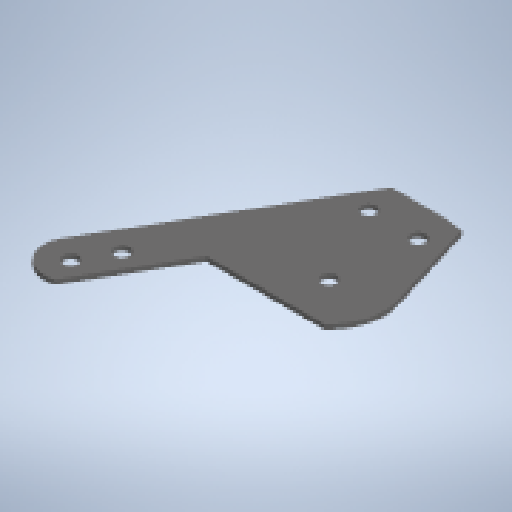
# Autodesk Inventor part: screw_cover_upper
Saved by Autodesk Inventor 2024.1 (Build 281209000, 209)
## iProperties
Created: 2025-01-18
Part Number: screw_cover_upper
Material: 一般
Document SubType Name: Modeling
Designer: hibik
Density: 1 g/cm^3
Appearance: 既定
Author: hibik
Autodesk Inventor part; units mm, degrees
ref_plane "YZ Plane" through (0, 0, 0) normal (1, 0, 0) x (0, 1, 0)
ref_plane "XZ Plane" through (0, 0, 0) normal (0, 1, 0) x (-1, 0, 0)
sketch "スケッチ1" plane through (0, 0, 0) normal (0, 1, 0) x (-1, 0, 0)
  circle A0 centre (0, 0) radius 8.9
  line L0 (0, -8.9) -> (63.2748, -8.9)
  line L1 (63.2748, -8.9) -> (63.2748, 8.9)
  line L2 (63.2748, 8.9) -> (0, 8.9)
  line L3 (0, 8.9) -> (0, -8.9)
  circle A1 centre (0, 0) radius 8.4
  line L4 (0, -8.4) -> (63.2748, -8.4)
  line L5 (63.2748, -8.4) -> (63.2748, 8.4)
  line L6 (63.2748, 8.4) -> (0, 8.4)
  line L7 (0, 8.4) -> (0, -8.4)
  point P0 (0, 8.4)
  point P1 (0, 8.9)
  dimension "d0" = 17.8
  dimension "d1" = 16.8
  constraints: 16 end point, 6 horizontal, 4 parallel, 3 coincident, 2 perpendicular, 1 collinear, 6 other
extrude "押し出し1" add sketch "スケッチ1" along normal blind 0.85 contours L3 A1 A0 | L2 L1 L6 A0 | A0 L6 L3 | L3 L4 A0 | A0 L4 L1 L0
sketch "スケッチ2" plane through (0, 0.85, 0) normal (0, 1, 0) x (1, 0, 0)
  circle A0 centre (0, 0) radius 12
  line L0 (0, 12) -> (-63.2748, 12)
  line L1 (-63.2748, 12) -> (-63.2748, -12)
  line L2 (-63.2748, -12) -> (0, -12)
  line L3 (0, -12) -> (0, 12)
  line L4 (-63.2748, 8.9) -> (-63.2748, 8.4) projected
  line L5 (-63.2748, 8.4) -> (0, 8.4) projected
  line L6 (0, -8.4) -> (-63.2748, -8.4) projected
  arc A1 (0, -8.4) -> (0, 8.4) centre (0, 0) ccw projected
  point P0 (0, -12)
  dimension "d4" = 24
  constraints: 8 end point, 3 horizontal, 2 parallel, 1 coincident, 1 collinear, 1 perpendicular, 3 other
extrude "押し出し2" add sketch "スケッチ2" along normal blind 1 contours A0 L3 A1 | L3 L5 A0 | A0 L5 L1 L0 | L2 L1 L6 A0 | A0 L6 L3
mirror "ミラー1" about plane through (-27.1874, 0, 0) normal (0, -1, 0)
sketch "スケッチ3" plane through (0, 1.85, 0) normal (0, 1, 0) x (1, 0, 0)
  line L0 (-14.7409, 17.0236) -> (-35.8476, -19.5343) projected
  line L1 (0, -8.4) -> (-63.2748, -8.4) projected
  line L2 (-63.2748, -8.4) -> (-63.2748, -12) projected
  line L3 (-63.2748, -12) -> (0, -12) projected
  arc A0 (0, -12) -> (0, 12) centre (0, 0) ccw projected
  line L4 (0, 12) -> (-63.2748, 12) projected
  line L5 (-63.2748, 12) -> (-63.2748, 8.4) projected
  line L6 (-63.2748, 8.4) -> (0, 8.4) projected
  arc A1 (0, -8.4) -> (0, 8.4) centre (0, 0) ccw projected
  point P0 (-31.4977, -12)
  point P1 (-29.4192, -8.4)
  point P2 (-19.7197, 8.4)
  point P3 (-17.6412, 12)
extrude "押し出し3" cut sketch "スケッチ3" against normal through all contours L0 L6 L5 L4 | L0 L3 L2 L1
ref_plane "作業平面1" through (0, -0.65, 0) normal (0, 1, 0) x (1, 0, 0)
sketch "スケッチ4" plane through (0, -0.65, 0) normal (0, 1, 0) x (1, 0, 0)
  line L0 (-19.7197, 8.4) -> (0, 8.4) projected
  arc A0 (0, -8.4) -> (0, 8.4) centre (0, 0) ccw projected
  line L1 (0, -8.4) -> (-29.4192, -8.4) projected
  line L2 (-19.7197, 8.4) -> (-29.4192, -8.4)
  circle A1 centre (0, 0) radius 1.6
  dimension "d10" = 3.2
  constraints: 2 coincident, 2 end point, 1 centre point
  measures "d10" diameter of A1
extrude "押し出し4" add sketch "スケッチ4" along normal up to surface (2.5 mm away)
fillet "フィレット1" radius 1 3 edges at (-9.8599, -0.65, -8.4) (8.4, -0.65, 0) (-14.7096, -0.65, 8.4)
sketch "スケッチ5" plane through (0, 1.85, 0) normal (0, 1, 0) x (1, 0, 0)
  circle A0 centre (-27.8315, -17.35) radius 1.6 projected
  circle A1 centre (-8.7282, 17.4379) radius 1.6 projected
  line L0 (0, 12) -> (-17.6412, 12) projected
  line L1 (-17.6412, 12) -> (-10.5885, 24.2158)
  line L2 (-10.5885, 24.2158) -> (0, 24.2158)
  line L3 (-39.933, -26.6105) -> (-10.6554, 24.0998) projected
  line L4 (0, 12) -> (-17.6412, 12) projected
  circle A2 centre (0, 0) radius 24.2158
  arc A3 (0, -12) -> (0, 12) centre (0, 0) ccw projected
  line L5 (11.4695, 3.5285) -> (5.2849, 23.6321)
  circle A4 centre (1.9592, 17.4379) radius 1.6
  line L6 (-39.933, -26.6105) -> (-10.6554, 24.0998) projected
  circle A5 centre (-31.9338, -24.4553) radius 1.6 projected
  circle A6 centre (-36, -34.6362) radius 1.6 projected
  circle A7 centre (-27.8315, -17.35) radius 1.6 projected
  line L7 (-39.933, -26.6105) -> (-10.6554, 24.0998) projected
  line L8 (-40, -50) -> (-40, -26.8605) projected
  line L9 (-38, -50.5) -> (-39.5, -50.5) projected
  line L10 (-31, -42) -> (-31, -32.0566) projected
  line L11 (-30.933, -31.8066) -> (-18.1986, -9.75) projected
  line L12 (-37.5, -50) -> (-37.5, -43) projected
  line L13 (-37, -42.5) -> (-31.5, -42.5) projected
  circle A8 centre (-31.9338, -24.4553) radius 5.85
  arc A9 (19.2639, -16.134) -> (19.9469, -15.951) centre (19.5139, -15.701) ccw projected
  line L14 (29.8557, 1.2115) -> (19.9469, -15.951) projected
  arc A10 (29.8557, 1.2115) -> (29.8557, 1.7115) centre (29.4226, 1.4615) ccw projected
  line L15 (10.25, 35.6695) -> (29.8557, 1.7115) projected
  arc A11 (10.25, 35.6695) -> (9.567, 35.8525) centre (9.817, 35.4195) ccw projected
  line L16 (-10.4724, 24.2828) -> (9.567, 35.8525) projected
  arc A12 (-10.4724, 24.2828) -> (-10.6554, 24.0998) centre (-10.2224, 23.8498) ccw projected
  arc A13 (-39.933, -26.6105) -> (-40, -26.8605) centre (-39.5, -26.8605) ccw projected
  arc A14 (-40, -50) -> (-39.5, -50.5) centre (-39.5, -50) ccw projected
  arc A15 (-38, -50.5) -> (-37.5, -50) centre (-38, -50) ccw projected
  arc A16 (-37, -42.5) -> (-37.5, -43) centre (-37, -43) ccw projected
  arc A17 (-31.5, -42.5) -> (-31, -42) centre (-31.5, -42) ccw projected
  arc A18 (-30.933, -31.8066) -> (-31, -32.0566) centre (-30.5, -32.0566) ccw projected
  arc A19 (-17.7656, -9.5) -> (-18.1986, -9.75) centre (-17.7656, -10) ccw projected
  line L17 (-17.7656, -9.5) -> (7.6395, -9.5) projected
  arc A20 (7.8895, -9.567) -> (7.6395, -9.5) centre (7.6395, -10) ccw projected
  line L18 (7.8895, -9.567) -> (19.2639, -16.134) projected
  circle A21 centre (1.9592, 17.4379) radius 1.6 projected
  circle A22 centre (24.5152, 1.2615) radius 1.6 projected
  circle A23 centre (5.1388, 27.5224) radius 1.6 projected
  circle A24 centre (13.1994, 17.561) radius 1.6 projected
  circle A25 centre (20.4199, -5.8317) radius 1.6 projected
  circle A26 centre (-8.7282, 17.4379) radius 1.6 projected
  circle A27 centre (0, 0) radius 1.5 projected
  point P0 (0, 24.2158)
  point P1 (-20.2427, -13.2905)
  point P2 (-12.6465, 20.6512)
  point P3 (-37, -21.5303)
  point P4 (-29.8432, -29.9191)
  point P5 (-26.1568, -23.5339)
  dimension "d14" = 15
  dimension "d15" = 3.2
  dimension "d16" = 5
  constraints: 4 end point, 3 centre point, 3 point on circle, 2 coincident, 2 tangent, 1 collinear, 1 horizontal, 1 horizontal alignment, 5 other
  measures "d14" distance from line of L1.end L5
  measures "d15" diameter of A4
  measures "d16" distance from line of L5 A4.centre
extrude "押し出し5" add sketch "スケッチ5" against normal blind 1 contours A1 | A3 L17 A19 L11 A2 L3 L0 | L0 L1 A2 L5 A3 | L5 A2 A22 L18 A20 L17 A3 | L1 A12 L2 A2 | A2 L11 A8 L3 | A2 L2 A12 L16 A11 L15 A10 L14 A9 L18 A22 | L1 L2 A12 | A8 L11 A18 L10 A17 L13 A16 L12 A15 L9 A14 L8 A13 L3 | A8 L11 | A22 A2 | A2 A22 | A8 L11 | A4 | A6 | A23 | A24 | A25 | A27
sketch "スケッチ6" plane through (0, 1.85, 0) normal (0, 1, 0) x (1, 0, 0)
  line L0 (-19.4977, -12) -> (0, -12) projected
  line L1 (-19.4977, -12) -> (-17.7656, -9)
  line L2 (-17.7656, -9) -> (7.9373, -9)
  arc A0 (0, -12) -> (0, 12) centre (0, 0) ccw projected
  line L3 (-29.8432, -29.9191) -> (-19.4977, -12) projected
  point P0 (-25.741, -22.8137)
  point P1 (-20.2427, -13.2905)
  point P2 (-31, -31.9226)
  dimension "d19" = 3
  constraints: 4 end point, 1 collinear, 1 parallel, 1 point on circle
  measures "d19" distance between parallel lines of L2 L0
extrude "押し出し6" cut sketch "スケッチ6" against normal through all
sketch "スケッチ7" plane through (0, -1.85, 0) normal (0, -1, 0) x (1, 0, 0)
  line L0 (-19.3733, -9) -> (0, -9) projected
  line L1 (-17.7656, 9) -> (-19.4977, 12) projected
  line L2 (-31.4977, 12) -> (-19.4977, 12) projected
  line L3 (-31.4977, 12) -> (-29.4192, 8.4) projected
  line L4 (0, 8.4) -> (-29.4192, 8.4) projected
  arc A0 (0, -8.4) -> (0, 8.4) centre (0, 0) ccw projected
  line L5 (-19.7197, -8.4) -> (0, -8.4) projected
  line L6 (-19.7197, -8.4) -> (-17.6412, -12) projected
  line L7 (0, -12) -> (-17.6412, -12) projected
  arc A1 (0, -12) -> (7.9373, 9) centre (0, 0) ccw projected
  line L8 (7.9373, 9) -> (-17.7656, 9) projected
  circle A2 centre (0, 0) radius 1.6 projected
  line L9 (0, -7.4) -> (-20.2971, -7.4) projected
  arc A3 (0, -7.4) -> (0, 7.4) centre (0, 0) ccw projected
  line L10 (-28.8418, 7.4) -> (0, 7.4) projected
  line L11 (-20.2971, -7.4) -> (-28.8418, 7.4) projected
  circle A4 centre (0, 0) radius 9 projected
  line L12 (-17.7656, 9) -> (7.9373, 9) projected
  line L13 (-10.5631, -24.2158) -> (-10.5885, -24.2158) projected
  arc A5 (-26.1568, 23.5339) -> (-29.8432, 29.9191) centre (-31.9338, 24.4553) ccw projected
  line L14 (-26.1568, 23.5339) -> (-17.7656, 9) projected
  circle A6 centre (-27.8315, 17.35) radius 1.6 projected
  circle A7 centre (-31.9338, 24.4553) radius 1.6 projected
  arc A8 (7.9373, 9) -> (7.3314, 9.5) centre (0, 0) ccw projected
  line L15 (7.3314, 9.5) -> (7.6395, 9.5) projected
  arc A9 (7.6395, 9.5) -> (7.8895, 9.567) centre (7.6395, 10) ccw projected
  line L16 (7.8895, 9.567) -> (19.2639, 16.134) projected
  arc A10 (19.9469, 15.951) -> (19.2639, 16.134) centre (19.5139, 15.701) ccw projected
  line L17 (19.9469, 15.951) -> (29.8557, -1.2115) projected
  arc A11 (29.8557, -1.7115) -> (29.8557, -1.2115) centre (29.4226, -1.4615) ccw projected
  line L18 (29.8557, -1.7115) -> (10.25, -35.6695) projected
  arc A12 (9.567, -35.8525) -> (10.25, -35.6695) centre (9.817, -35.4195) ccw projected
  line L19 (9.567, -35.8525) -> (-10.4724, -24.2828) projected
  arc A13 (-10.5631, -24.2158) -> (-10.4724, -24.2828) centre (-10.2224, -23.8498) ccw projected
  line L20 (-10.5885, -24.2158) -> (-39.933, 26.6105) projected
  arc A14 (-40, 26.8605) -> (-39.933, 26.6105) centre (-39.5, 26.8605) ccw projected
  line L21 (-40, 26.8605) -> (-40, 50) projected
  arc A15 (-39.5, 50.5) -> (-40, 50) centre (-39.5, 50) ccw projected
  line L22 (-39.5, 50.5) -> (-38, 50.5) projected
  arc A16 (-37.5, 50) -> (-38, 50.5) centre (-38, 50) ccw projected
  line L23 (-37.5, 50) -> (-37.5, 43) projected
  arc A17 (-37.5, 43) -> (-37, 42.5) centre (-37, 43) ccw projected
  line L24 (-37, 42.5) -> (-31.5, 42.5) projected
  arc A18 (-31, 42) -> (-31.5, 42.5) centre (-31.5, 42) ccw projected
  line L25 (-31, 42) -> (-31, 32.0566) projected
  arc A19 (-31, 32.0566) -> (-30.933, 31.8066) centre (-30.5, 32.0566) ccw projected
  line L26 (-30.933, 31.8066) -> (-29.8432, 29.9191) projected
  constraints: 1 vertical alignment
extrude "押し出し7" cut sketch "スケッチ7" against normal up to surface (2.7 mm away) contours L6 L5 A4 L0 | L0 A4 L8 A1 L7 L6 | A4 L5 A0 L4 | L11 L10 A4 L9 | A4 L4 L3 L2 L1 L8 | A4 L10 A3 L9 | A2
